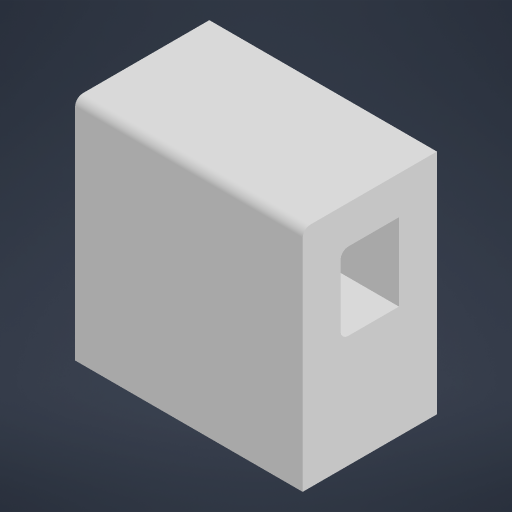
# Autodesk Inventor part: Clasp
Saved by Autodesk Inventor 2024.1 (Build 281209000, 209)
## iProperties
Created: 2023-09-06
Part Number: Clasp
Material: Generic
Document SubType Name: Modeling
Designer: User
Density: 1 g/cm^3
Appearance: Default
Author: User
Autodesk Inventor part; units mm, degrees
ref_plane "YZ Plane" through (0, 0, 0) normal (1, 0, 0) x (0, 1, 0)
ref_plane "XZ Plane" through (0, 0, 0) normal (0, 1, 0) x (-1, 0, 0)
ref_plane "XY Plane" through (0, 0, 0) normal (0, 0, 1) x (1, 0, 0)
sketch "Sketch5" plane through (0, 0, 0) normal (0, 0, 1) x (1, 0, 0)
  line L0 (0, 0) -> (-60, 0)
  line L1 (-60, 0) -> (-60, 60)
  line L2 (-60, 60) -> (0, 60)
  line L3 (0, 60) -> (0, 0)
  dimension "d55" = 60
  dimension "d56" = 60
  constraints: 8 end point, 2 parallel, 1 horizontal, 1 perpendicular
  measures "d55" distance of L1.end L2.end
  measures "d56" distance of L0.end L1.end
extrude "Extrusion4" add sketch "Sketch5" along normal blind 35.4
sketch "Sketch6" plane through (0, 0, 0) normal (1, 0, 0) x (0, 0, -1)
  line L0 (-35.4, 60) -> (-35.4, 0) projected
  line L1 (-35.4, 60) -> (-25.4, 60)
  line L2 (-25.4, 60) -> (-25.4, 50)
  line L3 (-25.4, 50) -> (-35.4, 50)
  line L4 (-35.4, 50) -> (-35.4, 60)
  line L5 (-25.4, 50) -> (-10, 50)
  line L6 (-10, 50) -> (-10, 29.6)
  line L7 (-10, 29.6) -> (-25.4, 29.6)
  line L8 (-25.4, 29.6) -> (-25.4, 50)
  point P0 (0, 0)
  dimension "d61" = 10
  dimension "d62" = 10
  dimension "d65" = 15.4
  dimension "d66" = 20.4
  constraints: 16 end point, 4 parallel, 2 horizontal, 2 perpendicular
  measures "d61" distance of L2.end L3.end
  measures "d62" distance of L1.end L2.end
  measures "d65" distance of L6.end L7.end
  measures "d66" distance of L5.end L6.end
extrude "Extrusion5" cut sketch "Sketch6" against normal blind 50 contours L5 L6 L7 L8
fillet "Fillet5" radius 2 3 edges at (-30, 60, 35.4) (-25, 29.6, 25.4) (-25, 50, 25.4)
body "Solid2"
